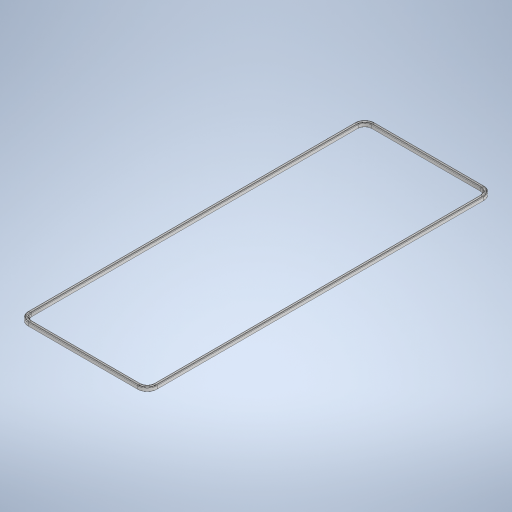
# Autodesk Inventor part: LI0005-SEAL
Saved by Autodesk Inventor 2023 (Build 270158000, 158)
## iProperties
Created: 2023-03-15
Part Number: LI0005-SEAL
Material: Generic
Document SubType Name: Modeling
Designer: Louis
Density: 1 g/cm^3
Appearance: Default
Author: Louis
Autodesk Inventor part; units mm, degrees
ref_plane "YZ Plane" through (0, 0, 0) normal (1, 0, 0) x (0, 1, 0)
ref_plane "XZ Plane" through (0, 0, 0) normal (0, 1, 0) x (-1, 0, 0)
ref_plane "XY Plane" through (0, 0, 0) normal (0, 0, 1) x (1, 0, 0)
sketch "Sketch1" plane through (0, 0, 0) normal (0, 1, 0) x (-1, 0, 0)
  circle A0 centre (65, 195) radius 12
  circle A1 centre (65, -195) radius 12
  circle A2 centre (-65, 195) radius 12
  circle A3 centre (-65, -195) radius 12
  line L0 (77, 195) -> (77, -195)
  line L1 (65, -207) -> (-65, -207)
  line L2 (65, 207) -> (-65, 207)
  line L3 (-77, 195) -> (-77, -195)
  line L4 (73, 195) -> (73, -195)
  circle A4 centre (65, 195) radius 8
  line L5 (65, 203) -> (-65, 203)
  circle A5 centre (-65, 195) radius 8
  line L6 (-73, 195) -> (-73, -195)
  circle A6 centre (-65, -195) radius 8
  line L7 (65, -203) -> (-65, -203)
  circle A7 centre (65, -195) radius 8
  point P0 (0, 0)
  point P1 (77, 0)
  point P2 (0, 207)
  point P3 (35, 143)
  point P4 (68, 135)
  point P5 (68, -135)
  point P6 (35, -143)
  point P7 (-60, -203)
  point P8 (-68, -135)
  point P9 (-68, 135)
  point P10 (-60, 203)
  dimension "d0" = 24
  dimension "d1" = 24
  dimension "d2" = 24
  dimension "d3" = 24
  dimension "d6" = 4
  dimension "d7" = 4
  dimension "d8" = 4
  dimension "d9" = 4
  dimension "d10" = 4
  dimension "d11" = 4
  dimension "d12" = 4
  dimension "d13" = 4
  dimension "d35" = 414
  dimension "d36" = 154
  constraints: 16 end point, 16 point on circle, 8 centre point, 6 parallel, 6 tangent, 3 horizontal alignment, 3 vertical alignment, 2 midpoint
  measures "d0" diameter of A0
  measures "d1" diameter of A2
  measures "d2" diameter of A1
  measures "d3" diameter of A3
  measures "d6" distance between parallel lines of L0 L4
  measures "d7" radial gap between concentric circles of A0 A4
  measures "d8" distance between parallel lines of L2 L5
  measures "d9" radial gap between concentric circles of A2 A5
  measures "d10" distance between parallel lines of L3 L6
  measures "d11" radial gap between concentric circles of A3 A6
  measures "d12" distance between parallel lines of L1 L7
  measures "d13" radial gap between concentric circles of A1 A7
  measures "d35" distance between parallel lines of L1 L2
  measures "d36" distance between parallel lines of L3 L0
extrude "Extrusion1" add sketch "Sketch1" along normal blind 4.5 contours A0 L4 A4 L5 | L0 A1 L4 A0 | A0 L5 A2 L2 | A1 L7 A7 L4 | A2 L5 A5 L6 | L1 A3 L7 A1 | A2 L6 A3 L3 | A3 L6 A6 L7 picked at (59.6594, 203.5636) picked at (59.6594, -203.5636) picked at (-59.6594, 203.5636) picked at (-59.6594, -203.5636)
sketch "Sketch2" plane through (0, 4.5, 0) normal (0, 1, 0) x (1, 0, 0)
  line L0 (-77, 195) -> (-77, -195) projected
  arc A0 (-77, -195) -> (-65, -207) centre (-65, -195) ccw projected
  line L1 (-65, -207) -> (65, -207) projected
  arc A1 (65, -207) -> (77, -195) centre (65, -195) ccw projected
  line L2 (77, -195) -> (77, 195) projected
  arc A2 (77, 195) -> (65, 207) centre (65, 195) ccw projected
  line L3 (65, 207) -> (-65, 207) projected
  arc A3 (-65, 207) -> (-77, 195) centre (-65, 195) ccw projected
  line L4 (-74.5, -195) -> (-74.5, 195)
  arc A4 (-65, 204.5) -> (-74.5, 195) centre (-65, 195) ccw
  line L5 (-65, 204.5) -> (65, 204.5)
  arc A5 (74.5, 195) -> (65, 204.5) centre (65, 195) ccw
  line L6 (74.5, 195) -> (74.5, -195)
  arc A6 (65, -204.5) -> (74.5, -195) centre (65, -195) ccw
  line L7 (65, -204.5) -> (-65, -204.5)
  arc A7 (-74.5, -195) -> (-65, -204.5) centre (-65, -195) ccw
  line L8 (-75.5, -195) -> (-75.5, 195)
  arc A8 (-65, 205.5) -> (-75.5, 195) centre (-65, 195) ccw
  line L9 (-65, 205.5) -> (65, 205.5)
  arc A9 (75.5, 195) -> (65, 205.5) centre (65, 195) ccw
  line L10 (75.5, 195) -> (75.5, -195)
  arc A10 (65, -205.5) -> (75.5, -195) centre (65, -195) ccw
  line L11 (65, -205.5) -> (-65, -205.5)
  arc A11 (-75.5, -195) -> (-65, -205.5) centre (-65, -195) ccw
  point P0 (0, 0)
  dimension "d16" = 2.5
  dimension "d17" = 1.5
  constraints: 16 end point, 16 point on circle, 8 centre point, 14 other
  measures "d16" distance between parallel lines of L0 L4
  measures "d17" distance between parallel lines of L0 L8
extrude "Extrusion2" cut sketch "Sketch2" against normal blind 1 contours L8 A8 L9 A9 L10 A10 L11 A11
chamfer "Chamfer3" distance 0.5 distance2 1 8 edges at (0, 4.5, 205.5) (-72.4246, 4.5, 202.4246) (-75.5, 4.5, 0) (-72.4246, 4.5, -202.4246) (0, 4.5, -205.5) (72.4246, 4.5, -202.4246) (75.5, 4.5, 0) (72.4246, 4.5, 202.4246) measured on face at (76, 4.5, -65)
chamfer "Chamfer4" distance 0.5 distance2 1 8 edges at (0, 4.5, 204.5) (71.7175, 4.5, 201.7175) (74.5, 4.5, 0) (71.7175, 4.5, -201.7175) (0, 4.5, -204.5) (-71.7175, 4.5, -201.7175) (-74.5, 4.5, 0) (-71.7175, 4.5, 201.7175) measured on face at (-74, 4.5, -65)
chamfer "Chamfer5" distance 0.5 angle 45 32 edges at (0, 4.5, 207) (73.4853, 4.5, 203.4853) (77, 4.5, 0) (73.4853, 4.5, -203.4853) (0, 4.5, -207) (-73.4853, 4.5, -203.4853) (-77, 4.5, 0) (-73.4853, 4.5, 203.4853) (0, 4.5, 203) (-70.6569, 4.5, 200.6569) (-73, 4.5, 0) (-70.6569, 4.5, -200.6569) (0, 4.5, -203) (70.6569, 4.5, -200.6569) (73, 4.5, 0) (70.6569, 4.5, 200.6569) (73.4853, 0, 203.4853) (77, 0, 0) (73.4853, 0, -203.4853) (0, 0, -207) (-73.4853, 0, -203.4853) (-77, 0, 0) (-73.4853, 0, 203.4853) (0, 0, 207) (0, 0, 203) (-70.6569, 0, 200.6569) (-73, 0, 0) (-70.6569, 0, -200.6569) (0, 0, -203) (70.6569, 0, -200.6569) (73, 0, 0) (70.6569, 0, 200.6569)
body "Solid1"
